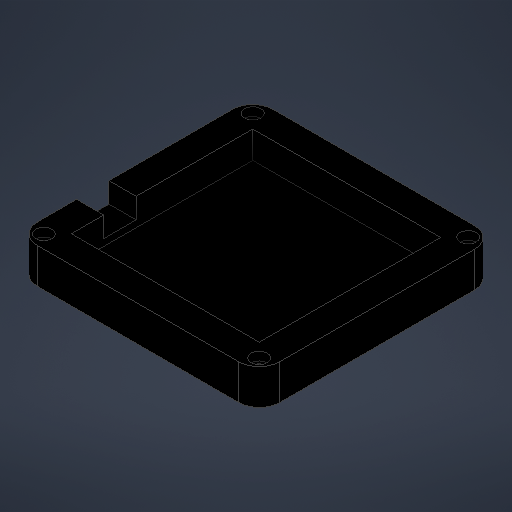
# Autodesk Inventor part: case bottom
Saved by Autodesk Inventor 2026 (Build 300175050, 175E)
## iProperties
Created: 2025-06-25
Part Number: case bottom
Material: Generic
Document SubType Name: Modeling
Designer: shlinke
Density: 1 g/cm^3
Appearance: Default
Author: shlinke
Autodesk Inventor part; units mm, degrees
ref_plane "YZ Plane" through (0, 0, 0) normal (1, 0, 0) x (0, 1, 0)
ref_plane "XZ Plane" through (0, 0, 0) normal (0, 1, 0) x (-1, 0, 0)
ref_plane "XY Plane" through (0, 0, 0) normal (0, 0, 1) x (1, 0, 0)
sketch "Sketch2" plane through (0, 0, 0) normal (0, 1, 0) x (-1, 0, 0)
  line L0 (34.528, 33.3375) -> (-34.528, 33.3375)
  line L1 (-34.528, 33.3375) -> (-34.528, -33.3375)
  line L2 (-34.528, -33.3375) -> (34.528, -33.3375)
  line L3 (34.528, -33.3375) -> (34.528, 33.3375)
  line L4 (34.528, 33.3375) -> (-34.528, -33.3375) construction
  line L5 (-34.528, 33.3375) -> (34.528, -33.3375) construction
  line L6 (44.528, -43.3375) -> (-44.528, -43.3375)
  line L7 (-44.528, -43.3375) -> (-44.528, 43.3375)
  line L8 (-44.528, 43.3375) -> (44.528, 43.3375)
  line L9 (44.528, 43.3375) -> (44.528, -43.3375)
  line L10 (44.528, -43.3375) -> (-44.528, 43.3375) construction
  line L11 (-44.528, -43.3375) -> (44.528, 43.3375) construction
  circle A0 centre (39.528, -38.3375) radius 1.7
  circle A1 centre (39.528, 38.4712) radius 1.7
  circle A2 centre (-39.528, -38.4712) radius 1.7
  circle A3 centre (-39.528, 38.3375) radius 1.7
  circle A4 centre (-39.528, -38.4712) radius 3
  circle A5 centre (-39.528, 38.3375) radius 3
  circle A6 centre (39.528, 38.4712) radius 3
  circle A7 centre (39.528, -38.3375) radius 3
  line L12 (34.528, 33.3375) -> (-34.528, 33.3375)
  line L13 (-34.528, 33.3375) -> (-34.528, -33.3375)
  line L14 (-34.528, -33.3375) -> (34.528, -33.3375)
  line L15 (34.528, -33.3375) -> (34.528, 33.3375)
  line L16 (34.528, 33.3375) -> (-34.528, -33.3375) construction
  line L17 (-34.528, 33.3375) -> (34.528, -33.3375) construction
  point P0 (0, 0)
  dimension "d1" = 66.675
  dimension "d2" = 69.056
  dimension "d3" = 10
  dimension "d4" = 10
  dimension "d6" = 5
  dimension "d7" = 5
  dimension "d8" = 3.4
  dimension "d9" = 5
  dimension "d10" = 3.4
  dimension "d11" = 5
  dimension "d12" = 3.4
  dimension "d13" = 3.4
  dimension "d14" = 5
  dimension "d15" = 5
  dimension "d16" = 6
  dimension "d17" = 6
  dimension "d18" = 6
  dimension "d19" = 6
  constraints: 36 end point, 8 centre point, 6 midpoint, 6 parallel, 4 coincident, 3 horizontal, 3 perpendicular, 2 point on line
  measures "d1" distance of L2.end L0.start
  measures "d2" distance of L1.end L2.end
  measures "d3" distance between parallel lines of L8 L0
  measures "d4" distance between parallel lines of L7 L1
  measures "d6" distance from line of L6 A0.centre
  measures "d7" distance from line of L9 A0.centre
  measures "d8" diameter of A1
  measures "d9" distance from line of L9 A1.centre
  measures "d10" diameter of A2
  measures "d11" distance from line of L7 A2.centre
  measures "d12" diameter of A0
  measures "d13" diameter of A3
  measures "d14" distance from line of L7 A3.centre
  measures "d15" distance from line of L8 A3.centre
  measures "d16" diameter of A4
  measures "d17" diameter of A5
  measures "d18" diameter of A6
  measures "d19" diameter of A7
extrude "Extrusion1" add sketch "Sketch2" along normal blind 13 contours L6 L7 L8 L9
extrude "Extrusion2" add sketch "Sketch2" along normal blind 3 contours L3 L2 L1 L0
extrude "Extrusion5" add sketch "Sketch2" along normal blind 9.9 contours A4 | A5 | A6 | A7
sketch "Sketch3" plane through (0, 13, 0) normal (0, 1, 0) x (1, 0, 0)
  line L0 (-34.528, -33.3375) -> (-34.528, 33.3375) construction
  line L1 (-34.528, -33.3375) -> (-44.528, -33.3375) construction
  line L2 (-44.528, 43.3375) -> (-44.528, -43.3375) construction
  line L3 (-39.528, -33.3375) -> (-39.528, -21.4315) construction
  line L4 (-44.528, -32.4315) -> (-44.528, -13.9315)
  line L5 (-34.528, -13.9315) -> (-34.528, -32.4315)
  line L6 (-34.528, -21.4315) -> (-52.0524, -21.4315)
  line L7 (-52.0524, -21.4315) -> (-52.0524, -9.5255)
  line L8 (-52.0524, -9.5255) -> (-34.528, -9.5255)
  line L9 (-34.528, -9.5255) -> (-34.528, -21.4315)
  point P0 (0, 0)
  dimension "d30" = 11.906
  dimension "d31" = 0
  dimension "d32" = 0
  dimension "d33" = 18.5
  dimension "d39" = 11.906
  constraints: 16 end point, 3 parallel, 2 horizontal, 2 point on line, 1 midpoint, 1 perpendicular, 1 vertical
  measures "d30" distance of L3.start L3.end
  measures "d31" distance between parallel lines of L2 L4
  measures "d32" distance between parallel lines of L0 L5
  measures "d33" distance of L5.start L5.end
  measures "d39" distance of L6.end L7.end
extrude "Extrusion6" cut sketch "Sketch3" against normal blind 7.5
fillet "Fillet1" radius 7.5 4 edges at (-44.528, 6.5, 43.3375) (44.528, 6.5, 43.3375) (44.528, 6.5, -43.3375) (-44.528, 6.5, -43.3375)
sketch "Sketch4" plane through (0, 0, 0) normal (0, -1, 0) x (1, 0, 0)
  line L0 (-43.474, -14.0672) -> (-43.474, 12.7577) construction
  line L1 (-43.474, 12.7577) -> (-42.3198, 12.7577) construction
  line L2 (-42.3198, 12.7577) -> (-42.3198, -14.0672) construction
  line L3 (-42.3198, -14.0672) -> (-43.474, -14.0672) construction
  line L4 (-40.2959, -13.8453) -> (-40.2959, -13.0189)
  line L5 (-40.2959, -13.0189) -> (-41.5712, -12.7944)
  spline S0 degree 2 poles (-41.5712, -12.7944) (-41.7676, -12.7562) (-41.9717, -12.5317) (-41.9717, -12.3761) knots 0 0 0 1 2 2 2
  spline S1 degree 2 poles (-41.9717, -12.3761) (-41.9717, -12.2205) (-41.7676, -12.0777) (-41.5712, -12.1109) knots 0 0 0 1 2 2 2
  line L6 (-41.5712, -12.1109) -> (-40.2959, -12.3353)
  line L7 (-40.2959, -12.3353) -> (-40.2959, -11.5115)
  line L8 (-40.2959, -11.5115) -> (-41.8365, -11.2411)
  spline S2 degree 2 poles (-41.8365, -11.2411) (-42.2446, -11.1697) (-42.6986, -11.5089) (-42.7037, -11.889) knots 0 0 0 1 2 2 2
  spline S3 degree 2 poles (-42.7037, -11.889) (-42.6986, -12.1389) (-42.4818, -12.5215) (-42.3288, -12.6618) knots 0 0 0 1 2 2 2
  line L9 (-42.3288, -12.6618) -> (-43.474, -12.4578)
  line L10 (-43.474, -12.4578) -> (-43.474, -13.2842)
  line L11 (-43.474, -13.2842) -> (-40.2959, -13.8453)
  spline S4 degree 2 poles (-40.2398, -9.8944) (-40.2449, -9.5143) (-40.5739, -8.869) (-41.13, -8.4354) (-41.4717, -8.3717) knots 0 0 0 1 2 3 3 3
  line L12 (-41.4717, -8.3717) -> (-41.4819, -8.3691)
  spline S5 degree 2 poles (-41.4819, -8.3691) (-41.8212, -8.313) (-42.3721, -8.5476) (-42.6986, -9.0731) (-42.7037, -9.4506) knots 0 0 0 1 2 3 3 3
  spline S6 degree 2 poles (-42.7037, -9.4506) (-42.6986, -9.8306) (-42.3696, -10.4759) (-41.8135, -10.907) (-41.4717, -10.9707) knots 0 0 0 1 2 3 3 3
  line L13 (-41.4717, -10.9707) -> (-41.4641, -10.9707)
  spline S7 degree 2 poles (-41.4641, -10.9707) (-41.1223, -11.0294) (-40.5714, -10.7947) (-40.2449, -10.2719) (-40.2398, -9.8944) knots 0 0 0 1 2 3 3 3
  spline S8 degree 2 poles (-40.9412, -9.7617) (-40.9463, -9.9836) (-41.2498, -10.2056) (-41.4717, -10.1698) knots 0 0 0 1 2 2 2
  line L14 (-41.4717, -10.1698) -> (-41.4819, -10.1673)
  spline S9 degree 2 poles (-41.4819, -10.1673) (-41.7039, -10.1265) (-42.0023, -9.8128) (-42.0074, -9.5832) knots 0 0 0 1 2 2 2
  spline S10 degree 2 poles (-42.0074, -9.5832) (-42.0023, -9.3587) (-41.6962, -9.1368) (-41.4717, -9.1725) knots 0 0 0 1 2 2 2
  line L15 (-41.4717, -9.1725) -> (-41.4641, -9.1725)
  spline S11 degree 2 poles (-41.4641, -9.1725) (-41.2447, -9.2134) (-40.9463, -9.5322) (-40.9412, -9.7617) knots 0 0 0 1 2 2 2
  line L16 (-40.2959, -8.2288) -> (-40.2959, -7.4024)
  line L17 (-40.2959, -7.4024) -> (-41.5763, -7.178)
  spline S12 degree 2 poles (-41.5763, -7.178) (-41.7727, -7.1397) (-41.9717, -6.9203) (-41.9717, -6.7724) knots 0 0 0 1 2 2 2
  spline S13 degree 2 poles (-41.9717, -6.7724) (-41.9717, -6.6245) (-41.7727, -6.4842) (-41.5763, -6.5148) knots 0 0 0 1 2 2 2
  line L18 (-41.5763, -6.5148) -> (-40.2959, -6.7418)
  line L19 (-40.2959, -6.7418) -> (-40.2959, -5.9179)
  line L20 (-40.2959, -5.9179) -> (-41.5763, -5.6935)
  spline S14 degree 2 poles (-41.5763, -5.6935) (-41.7727, -5.6552) (-41.9717, -5.4333) (-41.9717, -5.2828) knots 0 0 0 1 2 2 2
  spline S15 degree 2 poles (-41.9717, -5.2828) (-41.9717, -5.1349) (-41.7727, -4.9997) (-41.5763, -5.0303) knots 0 0 0 1 2 2 2
  line L21 (-41.5763, -5.0303) -> (-40.2959, -5.2573)
  line L22 (-40.2959, -5.2573) -> (-40.2959, -4.4309)
  line L23 (-40.2959, -4.4309) -> (-41.8416, -4.158)
  spline S16 degree 2 poles (-41.8416, -4.158) (-42.2573, -4.0891) (-42.7011, -4.4309) (-42.7037, -4.811) knots 0 0 0 1 2 2 2
  spline S17 degree 2 poles (-42.7037, -4.811) (-42.7011, -5.0686) (-42.5022, -5.4843) (-42.3211, -5.6654) knots 0 0 0 1 2 2 2
  spline S18 degree 2 poles (-42.3211, -5.6654) (-42.5047, -5.7292) (-42.7011, -6.0404) (-42.7037, -6.2776) knots 0 0 0 1 2 2 2
  spline S19 degree 2 poles (-42.7037, -6.2776) (-42.6986, -6.525) (-42.4818, -6.905) (-42.3288, -7.0453) knots 0 0 0 1 2 2 2
  line L24 (-42.3288, -7.0453) -> (-42.6501, -6.9867)
  line L25 (-42.6501, -6.9867) -> (-42.6501, -7.8131)
  line L26 (-42.6501, -7.8131) -> (-40.2959, -8.2288)
  spline S20 degree 2 poles (-40.2398, -2.8419) (-40.2423, -2.4899) (-40.4974, -1.9466) (-40.7168, -1.74) knots 0 0 0 1 2 2 2
  line L27 (-40.7168, -1.74) -> (-41.0968, -2.1303)
  spline S21 degree 2 poles (-41.0968, -2.1303) (-40.9693, -2.2757) (-40.857, -2.5435) (-40.857, -2.694) knots 0 0 0 1 2 2 2
  spline S22 degree 2 poles (-40.857, -2.694) (-40.857, -2.8904) (-41.0483, -3.1199) (-41.2447, -3.1352) knots 0 0 0 1 2 2 2
  line L28 (-41.2447, -3.1352) -> (-41.2447, -1.5589)
  spline S23 degree 2 poles (-41.2447, -1.5589) (-41.2881, -1.5487) (-41.3748, -1.5309) (-41.4156, -1.5258) knots 0 0 0 1 2 2 2
  spline S24 degree 2 poles (-41.4156, -1.5258) (-41.7651, -1.462) (-42.3466, -1.615) (-42.6986, -2.0793) (-42.7037, -2.4823) knots 0 0 0 1 2 3 3 3
  spline S25 degree 2 poles (-42.7037, -2.4823) (-42.6986, -2.8317) (-42.3721, -3.4234) (-41.8161, -3.8239) (-41.4717, -3.8876) knots 0 0 0 1 2 3 3 3
  line L29 (-41.4717, -3.8876) -> (-41.4641, -3.8876)
  spline S26 degree 2 poles (-41.4641, -3.8876) (-41.0968, -3.9514) (-40.5484, -3.727) (-40.2423, -3.2143) (-40.2398, -2.8419) knots 0 0 0 1 2 3 3 3
  spline S27 degree 2 poles (-41.6681, -3.074) (-41.8645, -3.0026) (-42.0915, -2.7552) (-42.0941, -2.5894) knots 0 0 0 1 2 2 2
  spline S28 degree 2 poles (-42.0941, -2.5894) (-42.0915, -2.4185) (-41.8645, -2.2399) (-41.6681, -2.2501) knots 0 0 0 1 2 2 2
  line L30 (-41.6681, -2.2501) -> (-41.6681, -3.074)
  line L31 (-40.2959, -1.3166) -> (-40.2959, -0.4724)
  line L32 (-40.2959, -0.4724) -> (-41.1682, -0.3193)
  line L33 (-41.1682, -0.3193) -> (-41.1682, 0.1041)
  spline S29 degree 2 poles (-41.1682, 0.1041) (-41.1682, 0.4841) (-41.4182, 1.1141) (-41.9079, 1.535) (-42.2701, 1.6013) knots 0 0 0 1 2 3 3 3
  line L34 (-42.2701, 1.6013) -> (-42.2777, 1.6039)
  spline S30 degree 2 poles (-42.2777, 1.6039) (-42.617, 1.6625) (-43.0914, 1.4355) (-43.3439, 0.9152) (-43.3439, 0.53) knots 0 0 0 1 2 3 3 3
  line L35 (-43.3439, 0.53) -> (-43.3439, -0.7784)
  line L36 (-43.3439, -0.7784) -> (-40.2959, -1.3166)
  line L37 (-41.8288, -0.202) -> (-42.6348, -0.0592)
  line L38 (-42.6348, -0.0592) -> (-42.6348, 0.3413)
  spline S31 degree 2 poles (-42.6348, 0.3413) (-42.6348, 0.5683) (-42.4359, 0.7902) (-42.2395, 0.757) knots 0 0 0 1 2 2 2
  line L39 (-42.2395, 0.757) -> (-42.2293, 0.757)
  spline S32 degree 2 poles (-42.2293, 0.757) (-42.0456, 0.7213) (-41.8314, 0.428) (-41.8288, 0.2036) knots 0 0 0 1 2 2 2
  line L40 (-41.8288, 0.2036) -> (-41.8288, -0.202)
  spline S33 degree 2 poles (-40.2423, 2.2288) (-40.2449, 2.4634) (-40.4056, 2.8307) (-40.5433, 2.9812) knots 0 0 0 1 2 2 2
  line L41 (-40.5433, 2.9812) -> (-40.2959, 2.9378)
  line L42 (-40.2959, 2.9378) -> (-40.2959, 3.7515)
  line L43 (-40.2959, 3.7515) -> (-41.6503, 3.9912)
  spline S34 degree 2 poles (-41.6503, 3.9912) (-41.8977, 4.0346) (-42.2701, 3.981) (-42.4002, 3.8688) knots 0 0 0 1 2 2 2
  spline S35 degree 2 poles (-42.4002, 3.8688) (-42.5405, 3.7566) (-42.6858, 3.3383) (-42.6858, 3.022) knots 0 0 0 1 2 2 2
  spline S36 degree 2 poles (-42.6858, 3.022) (-42.6833, 2.721) (-42.5864, 2.2466) (-42.5022, 2.0375) knots 0 0 0 1 2 2 2
  line L44 (-42.5022, 2.0375) -> (-41.9258, 2.1038)
  spline S37 degree 2 poles (-41.9258, 2.1038) (-41.987, 2.2721) (-42.0558, 2.596) (-42.0558, 2.7822) knots 0 0 0 1 2 2 2
  spline S38 degree 2 poles (-42.0558, 2.7822) (-42.0558, 3.0195) (-41.8543, 3.2184) (-41.6656, 3.1852) knots 0 0 0 1 2 2 2
  line L45 (-41.6656, 3.1852) -> (-41.6273, 3.1776)
  spline S39 degree 2 poles (-41.6273, 3.1776) (-41.6681, 3.0807) (-41.7192, 2.795) (-41.7192, 2.6267) knots 0 0 0 1 2 2 2
  spline S40 degree 2 poles (-41.7192, 2.6267) (-41.7192, 2.2058) (-41.3493, 1.6421) (-40.9795, 1.5707) knots 0 0 0 1 2 2 2
  line L46 (-40.9795, 1.5707) -> (-40.9718, 1.5707)
  spline S41 degree 2 poles (-40.9718, 1.5707) (-40.7372, 1.5299) (-40.4107, 1.6778) (-40.2423, 2.0043) (-40.2423, 2.2288) knots 0 0 0 1 2 3 3 3
  spline S42 degree 2 poles (-40.7627, 2.619) (-40.7627, 2.4889) (-40.8979, 2.3512) (-41.0177, 2.3716) knots 0 0 0 1 2 2 2
  line L47 (-41.0177, 2.3716) -> (-41.0279, 2.3716)
  spline S43 degree 2 poles (-41.0279, 2.3716) (-41.1631, 2.3971) (-41.3162, 2.619) (-41.3187, 2.8052) knots 0 0 0 1 2 2 2
  spline S44 degree 2 poles (-41.3187, 2.8052) (-41.3187, 2.897) (-41.2855, 3.0603) (-41.2575, 3.1215) knots 0 0 0 1 2 2 2
  line L48 (-41.2575, 3.1215) -> (-41.1504, 3.1011)
  spline S45 degree 2 poles (-41.1504, 3.1011) (-40.9693, 3.0654) (-40.7652, 2.8052) (-40.7627, 2.619) knots 0 0 0 1 2 2 2
  spline S46 degree 2 poles (-40.2423, 5.1212) (-40.2474, 5.3839) (-40.4566, 5.7563) (-40.6071, 5.9017) knots 0 0 0 1 2 2 2
  line L49 (-40.6071, 5.9017) -> (-40.2959, 5.8455)
  line L50 (-40.2959, 5.8455) -> (-40.2959, 6.672)
  line L51 (-40.2959, 6.672) -> (-43.474, 7.2331)
  line L52 (-43.474, 7.2331) -> (-43.474, 6.4067)
  line L53 (-43.474, 6.4067) -> (-42.3645, 6.2103)
  spline S47 degree 2 poles (-42.3645, 6.2103) (-42.5022, 6.1236) (-42.6986, 5.8124) (-42.7037, 5.5497) knots 0 0 0 1 2 2 2
  spline S48 degree 2 poles (-42.7037, 5.5497) (-42.7011, 5.2666) (-42.4053, 4.7462) (-41.8569, 4.3636) (-41.4717, 4.2922) knots 0 0 0 1 2 3 3 3
  line L54 (-41.4717, 4.2922) -> (-41.4615, 4.2922)
  spline S49 degree 2 poles (-41.4615, 4.2922) (-41.0841, 4.2284) (-40.5382, 4.4172) (-40.2449, 4.838) (-40.2423, 5.1212) knots 0 0 0 1 2 3 3 3
  spline S50 degree 2 poles (-40.9336, 5.491) (-40.9387, 5.2895) (-41.2294, 5.0651) (-41.4692, 5.1008) knots 0 0 0 1 2 2 2
  line L55 (-41.4692, 5.1008) -> (-41.4794, 5.1033)
  spline S51 degree 2 poles (-41.4794, 5.1033) (-41.6375, 5.1314) (-41.8773, 5.3074) (-42.015, 5.5497) (-42.015, 5.6823) knots 0 0 0 1 2 3 3 3
  spline S52 degree 2 poles (-42.015, 5.6823) (-42.0125, 5.8889) (-41.7192, 6.1083) (-41.4794, 6.0726) knots 0 0 0 1 2 2 2
  line L56 (-41.4794, 6.0726) -> (-41.4692, 6.07)
  spline S53 degree 2 poles (-41.4692, 6.07) (-41.2294, 6.0241) (-40.9387, 5.7002) (-40.9336, 5.491) knots 0 0 0 1 2 2 2
  line L57 (-40.2781, 9.1818) -> (-40.2781, 9.9342)
  line L58 (-40.2781, 9.9342) -> (-42.6501, 11.2937)
  line L59 (-42.6501, 11.2937) -> (-42.6501, 10.4392)
  line L60 (-42.6501, 10.4392) -> (-41.2753, 9.7404)
  line L61 (-41.2753, 9.7404) -> (-42.6501, 9.5287)
  line L62 (-42.6501, 9.5287) -> (-42.6501, 8.6589)
  line L63 (-42.6501, 8.6589) -> (-40.2781, 9.1818)
  line L64 (-40.2959, 11.6304) -> (-40.2959, 12.4619)
  line L65 (-40.2959, 12.4619) -> (-43.3669, 13.0026)
  line L66 (-43.3669, 13.0026) -> (-43.3669, 12.3905)
  line L67 (-43.3669, 12.3905) -> (-43.1143, 11.4518)
  line L68 (-43.1143, 11.4518) -> (-42.4614, 11.4977)
  line L69 (-42.4614, 11.4977) -> (-42.5838, 12.0334)
  line L70 (-42.5838, 12.0334) -> (-40.2959, 11.6304)
  point P0 (0, 0)
  dimension "d2" = 69.056
  constraints: 2 other
extrude "Extrusion7" cut sketch "Sketch4" against normal blind 0.2
body "Solid1"
